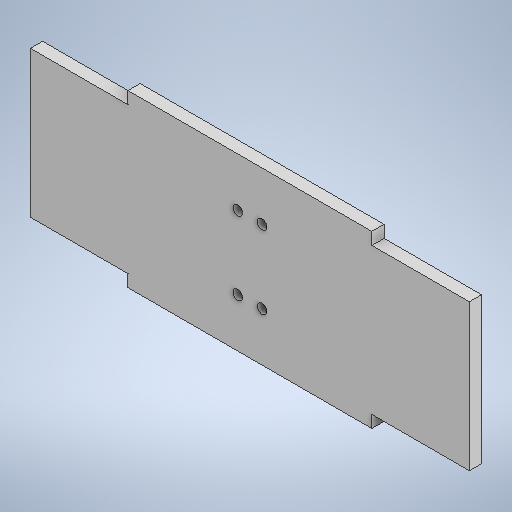
# Autodesk Inventor part: front
Saved by Autodesk Inventor 2025.3 (Build 293356030, 356C)
## iProperties
Created: 2026-06-26
Part Number: front
Material: Generic
Document SubType Name: Modeling
Designer: user
Density: 1 g/cm^3
Appearance: Default
Author: user
Autodesk Inventor part; units mm, degrees
ref_plane "YZ Plane" through (0, 0, 0) normal (1, 0, 0) x (0, 1, 0)
ref_plane "XZ Plane" through (0, 0, 0) normal (0, 1, 0) x (-1, 0, 0)
ref_plane "XY Plane" through (0, 0, 0) normal (0, 0, 1) x (1, 0, 0)
sketch "Sketch1" plane through (0, 0, 0) normal (0, 0, 1) x (1, 0, 0)
  line L0 (0, 0) -> (180, 0)
  line L1 (180, 0) -> (180, 60)
  line L2 (180, 60) -> (0, 60)
  line L3 (0, 60) -> (0, 0)
  line L4 (40, 0) -> (140, 0)
  line L5 (140, 0) -> (140, -5)
  line L6 (140, -5) -> (40, -5)
  line L7 (40, -5) -> (40, 0)
  line L8 (40, 60) -> (140, 60)
  line L9 (140, 60) -> (140, 65)
  line L10 (140, 65) -> (40, 65)
  line L11 (40, 65) -> (40, 60)
  point P0 (0, 20)
  point P1 (140, 0)
  point P2 (140, 60)
  point P3 (40, 62.5)
  dimension "d0" = 180
  dimension "d1" = 60
  dimension "d2" = 100
  dimension "d3" = 5
  dimension "d8" = 40
  dimension "d9" = 5
  dimension "d10" = 100
  dimension "d11" = 40
  constraints: 24 end point, 6 parallel, 3 horizontal, 3 perpendicular, 3 point on line, 1 midpoint
  measures "d0" distance of L2.end L1.end
  measures "d1" distance of L1.end L0.end
  measures "d2" distance of L5.end L6.end
  measures "d3" distance of L4.end L5.end
  measures "d8" distance from line of L7 L0.start
  measures "d9" distance of L9.end L8.end
  measures "d10" distance between parallel lines of L9 L11
  measures "d11" distance from line of point (40, 62.5) L3
extrude "Extrusion1" add sketch "Sketch1" along normal blind 5
sketch "Sketch3" plane through (0, 0, 5) normal (0, 0, 1) x (1, 0, 0)
  line L0 (140, 65) -> (40, 65) projected
  line L1 (40, -5) -> (140, -5) projected
  line L2 (40, 65) -> (40, 60) projected
  line L3 (40, 0) -> (40, -5) projected
  point P0 (0, 0)
  point P1 (85, 45)
  point P2 (95, 45)
  point P3 (85, 15)
  point P4 (95, 15)
  dimension "d19" = 20
  dimension "d20" = 20
  dimension "d21" = 20
  dimension "d22" = 20
  dimension "d23" = 10
  dimension "d24" = 10
  dimension "d25" = 45
  dimension "d26" = 45
  measures "d19" distance from line of L0 point (85, 45)
  measures "d20" distance from line of L1 point (85, 15)
  measures "d21" distance from line of L1 point (95, 15)
  measures "d22" distance from line of L0 point (95, 45)
  measures "d23" distance of point (95, 45) point (85, 45)
  measures "d24" distance of point (95, 15) point (85, 15)
  measures "d25" distance from line of point (85, 45) L2
  measures "d26" distance from line of point (85, 15) L3
hole "Hole1" at (85, 45, 5) at (95, 45, 5) at (85, 15, 5) at (95, 15, 5) direction (0, 0, -1) diameter 4 end through all
body "Solid1"
